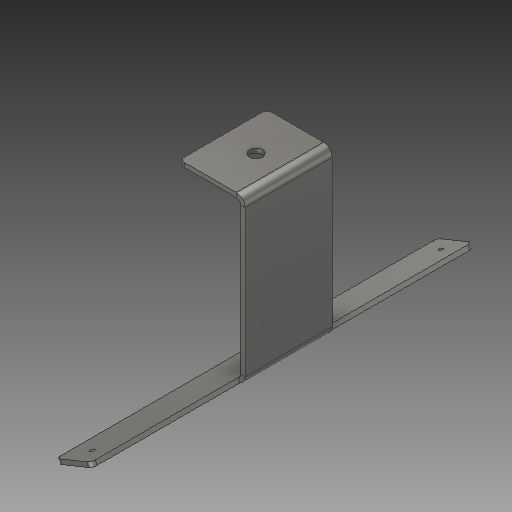
# Autodesk Inventor part: Bottom Mount
Saved by Autodesk Inventor 2019 (Build 230136000, 136)
## iProperties
Created: 2020-02-21
Part Number: Bottom Mount
Material: Stainless Steel
Document SubType Name: Sheet Metal
Designer: gfb14170
Density: 8 g/cm^3
Sheet Metal Rule: Default_mm
Appearance: Semi-Polished
Flat Pattern Width: 11.8546 cm
Flat Pattern Length: 17.5 cm
Flat Pattern Area: 207.455 cm^2
Sheet Metal Width: 118.546 mm
Sheet Metal Length: 175.000 mm
Sheet Metal Area: 20745.529 mm^2
Author: gfb14170
Autodesk Inventor part; units mm, degrees
ref_plane "YZ Plane" through (0, 0, 0) normal (1, 0, 0) x (0, 1, 0)
ref_plane "XZ Plane" through (0, 0, 0) normal (0, 1, 0) x (-1, 0, 0)
ref_plane "XY Plane" through (0, 0, 0) normal (0, 0, 1) x (1, 0, 0)
sketch "Sketch1" plane through (0, 0, 0) normal (0, 1, 0) x (-1, 0, 0)
  line L0 (0, 20) -> (-30, 20)
  line L1 (-30, 20) -> (-30, -20)
  line L2 (-30, -20) -> (0, -20)
  line L3 (0, -20) -> (0, 20)
  point P0 (0, 0)
  dimension "d0" = 20
  dimension "d1" = 20
  dimension "d2" = 0
  dimension "d3" = 30
  measures "d0" distance from line of L0 point (0, 0)
  measures "d1" distance from line of point (0, 0) L2
  measures "d2" distance from line of point (0, 0) L3
  measures "d3" distance from line of point (0, 0) L1
extrude "Plate1" add sketch "Sketch1" along normal blind 2
sketch "Sketch2" plane through (28, 2, -20) normal (1, 0, 0) x (0, -1, 0)
  line L0 (0, 40) -> (0, 0)
  line L1 (0, 0) -> (74, 0)
  line L2 (74, 0) -> (74, 40)
  line L3 (74, 40) -> (0, 40)
  constraints: 6 end point, 1 horizontal, 1 perpendicular, 1 vertical
edge flange "Flange1" height 74 angle -90 thickness 2 bend radius 2 thickness toward (1, 0, 0) relief straight relief width 2 relief depth 1 edges at (30, 2, 0) wall of the first edge with corners at (28, 2, 20) (28, 2, -20) (28, -72, -20) (28, -72, 20)
bend "Bend1"
corner "Corner1"
sketch "Sketch3" plane through (29.2508, -70.1456, 20) normal (0.3746066, -0.9271839, 0) x (0.9271839, 0.3746066, 0)
  line L0 (0, -40) -> (0, 0)
  line L1 (0, 0) -> (-20, 0)
  line L2 (-20, 0) -> (-20, -40)
  line L3 (-20, -40) -> (0, -40)
  constraints: 6 end point, 1 horizontal, 1 perpendicular, 1 vertical
edge flange "Flange2" height 20 angle 68 thickness 2 bend radius 2 thickness toward (0.3746066, -0.9271839, 0) relief straight relief width 2 relief depth 1 edges at (28, -72, 0) wall of the first edge with corners at (29.2508, -70.1456, -20) (29.2508, -70.1456, 20) (10.7071, -77.6378, 20) (10.7071, -77.6378, -20)
bend "Bend2"
corner "Corner2"
sketch "Sketch4" plane through (11.4563, -79.4921, 20) normal (0.3746066, -0.9271839, 0) x (-0.9271839, -0.3746066, 0)
  line L0 (-17.302, 40) -> (-17.302, 0) projected
  line L1 (0, 0) -> (-17.302, 0) projected
  line L2 (0, 40) -> (0, 0) projected
  line L3 (-17.302, 40) -> (0, 40) projected
  line L4 (-17.302, -67.5) -> (0, -67.5)
  line L5 (0, -67.5) -> (0, 107.5)
  line L6 (0, 107.5) -> (-17.302, 107.5)
  line L7 (-17.302, 107.5) -> (-17.302, -67.5)
  point P0 (-19.1562, 20)
  dimension "d26" = 87.5
  dimension "d27" = 87.5
  dimension "d28" = 0
  dimension "d30" = 0
  constraints: 8 end point, 2 parallel, 1 horizontal, 1 perpendicular
  measures "d26" distance from line of L4 point (-19.156, 20)
  measures "d27" distance from line of L6 point (-19.156, 20)
  measures "d28" distance between parallel lines of L0 L7
  measures "d30" distance between parallel lines of L2 L5
extrude "Extrusion1" add sketch "Sketch4" against normal blind 2 contours L7 L6 L5 L3 | L1 L5 L4 L7
sketch "Sketch5" plane through (0, 2, 0) normal (0, 1, 0) x (1, 0, 0)
  circle A0 centre (15, 0) radius 3
  line L0 (36, 0) -> (-6, 0) projected
  point P0 (0, 0)
  dimension "d51" = 6
  dimension "d52" = 0
  dimension "d53" = 15
  constraints: 1 centre point
  measures "d51" diameter of A0
  measures "d52" distance from line of L0 A0.centre
  measures "d53" distance of point (0, 0) A0.centre
extrude "Extrusion2" cut sketch "Sketch5" against normal blind 2
sketch "Sketch6" plane through (27.4984, -73.0107, 87.5) normal (0.3746066, -0.9271839, 0) x (-0.9271839, -0.3746066, 0)
  circle A0 centre (8, 8) radius 1
  line L0 (0, 107.5) -> (0, 67.5) projected
  line L1 (0, 67.5) -> (0, 0) projected
  line L2 (0, 0) -> (17.302, 0) projected
  line L3 (17.302, 0) -> (17.302, 175) projected
  line L4 (17.302, 175) -> (0, 175) projected
  line L5 (0, 175) -> (0, 107.5) projected
  circle A1 centre (8, 168) radius 1
  point P0 (-1.8542, 87.5)
  dimension "d38" = 2
  dimension "d39" = 8
  dimension "d40" = 8
  dimension "d43" = 160
  constraints: 2 centre point, 1 vertical, 2 other
  measures "d38" diameter of A0
  measures "d39" distance from line of L2 A0.centre
  measures "d40" distance from line of L1 A0.centre
  measures "d43" distance of A0.centre A1.centre
extrude "Extrusion3" cut sketch "Sketch6" against normal blind 2 contours A0 | A1
fillet "Fillet1" radius 2 6 edges at (0, 1, 20) (0, 1, -20) (11.0817, -78.5649, 87.5) (27.1238, -72.0835, 87.5) (11.0817, -78.5649, -87.5) (27.1238, -72.0835, -87.5)
equation "\"d4\" = Thickness"
equation "\"d5\" = BendReliefWidth"
equation "\"d6\" = BendReliefDepth"
equation "\"d7\" = MinimumRemnant"
equation "\"d8\" = TransitionRadius"
equation "\"d11\" = BendRadius"
equation "\"d12\" = CornerReliefSize"
equation "\"d13\" = GapSize"
equation "\"d14\" = JacobiRadiusSize"
equation "\"d15\" = BendReliefWidth"
equation "\"d16\" = BendReliefDepth"
equation "\"d17\" = MinimumRemnant"
equation "\"d18\" = TransitionRadius"
equation "\"d21\" = BendRadius"
equation "\"d22\" = CornerReliefSize"
equation "\"d23\" = GapSize"
equation "\"d24\" = JacobiRadiusSize"
equation "\"d27\" = d26"
equation "\"d1\" = d0"
equation "\"BendRadius\" = Thickness"
equation "\"BendReliefWidth\" = Thickness"
equation "\"BendReliefDepth\" = 0.5 * Thickness"
equation "\"CornerReliefSize\" = 4 * Thickness"
equation "\"MinimumRemnant\" = 2 * Thickness"
equation "\"TransitionRadius\" = BendRadius"
equation "\"JacobiRadiusSize\" = BendRadius"
equation "\"GapSize\" = Thickness"
equation "\"Thickness\" = 2"
body "Solid1"
